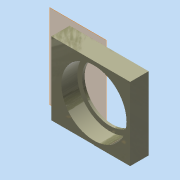
# Autodesk Inventor part: 10_Filteslide_25mm
Saved by Autodesk Inventor 2019.4 (Build 234330000, 330)
## iProperties
Created: 2019-08-26
Part Number: 10_Filteslide_25mm
Material: Generic
Document SubType Name: Modeling
Designer: diederichbenedict
Density: 1 g/cm^3
Appearance: Smooth - Ash
Author: diederichbenedict
Autodesk Inventor part; units mm, degrees
ref_plane "YZ Plane" through (0, 0, 0) normal (1, 0, 0) x (0, 1, 0)
ref_plane "XZ Plane" through (0, 0, 0) normal (0, 1, 0) x (-1, 0, 0)
ref_plane "XY Plane" through (0, 0, 0) normal (0, 0, 1) x (1, 0, 0)
ref_plane "Work Plane1" through (0, 0, 0) normal (0, 0, 1) x (1, 0, 0)
sketch "Sketch1" plane through (0, 0, 0) normal (0, 0, 1) x (1, 0, 0)
  arc A0 (-18.155, 30) -> (-18.155, 0) centre (0, 15) ccw construction
  line L0 (-18.155, 0) -> (-3.4871, 0) construction
  line L1 (-18.155, 30) -> (-3.4871, 30) construction
  circle A1 centre (0, 15) radius 15.4 construction
  line L2 (-6.5238, 0.75) -> (-17.7982, 0.75) construction
  line L3 (-17.7982, 29.25) -> (-6.5238, 29.25) construction
  line L4 (-6.5238, 29.25) -> (0, 29.25) construction
  line L5 (-6.5238, 0.75) -> (0, 0.75) construction
  line L6 (-16.7452, 29.25) -> (-16.7452, 0.75)
  line L7 (-16.7452, 0.75) -> (0, 0.75)
  line L8 (-16.7452, 29.25) -> (0, 29.25)
  arc A2 (-3.4871, 0) -> (3.4871, 0) centre (0, 15) ccw projected
  line L9 (3.4871, 0) -> (18, 0) projected
  line L10 (18, 0) -> (18, 30) projected
  line L11 (3.4871, 30) -> (18, 30) projected
  arc A3 (3.4871, 30) -> (-3.4871, 30) centre (0, 15) ccw projected
  line L12 (-7.3927, 28.5095) -> (7.3927, 28.5095) projected
  arc A4 (7.3927, 1.4905) -> (7.3927, 28.5095) centre (0, 15) ccw projected
  line L13 (7.3927, 1.4905) -> (-7.3927, 1.4905) projected
  arc A5 (-7.3927, 28.5095) -> (-7.3927, 1.4905) centre (0, 15) ccw projected
  line L14 (14.65, 3.6133) -> (14.65, -23.4854) projected
  line L15 (0, 29.25) -> (14.2, 29.25)
  line L16 (14.2, 29.25) -> (14.2, 0.6479)
  line L17 (14.2, 0.6479) -> (0, 0.6479)
  circle A6 centre (0, 15) radius 10.9034
  line L18 (0, 0.6479) -> (0, 0.75)
  point P0 (0, 0)
  dimension "d8" = 14.2
  constraints: 22 end point, 3 parallel, 2 perpendicular, 2 point on line, 1 centre point, 1 coincident, 1 horizontal, 1 vertical
  measures "d8" distance of L16.end L17.end
extrude "Extrusion1" add sketch "Sketch1" along normal blind 1 contours L8 L15 L16 A4 L12 A5 L13 L17 L18 L7 L6 | L16 A4 L13 A5 L12
sketch "Sketch2" plane through (0, 0, 1) normal (0, 0, 1) x (1, 0, 0)
  line L0 (14.2, 29.25) -> (-16.7452, 29.25) projected
  line L1 (-16.7452, 29.25) -> (-16.7452, 0.75) projected
  line L2 (-16.7452, 0.75) -> (0, 0.75) projected
  circle A0 centre (0, 15) radius 12.775
  line L3 (0, 0.75) -> (0, 0.6479) projected
  line L4 (0, 0.6479) -> (14.2, 0.6479) projected
  line L5 (14.2, 0.6479) -> (14.2, 29.25) projected
  point P0 (0, 0)
  dimension "d5" = 25.55
  constraints: 1 centre point
  measures "d5" diameter of A0
extrude "Extrusion2" add sketch "Sketch2" along normal blind 6.25
body "Solid1"
